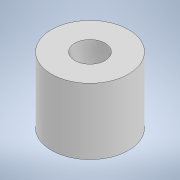
# Autodesk Inventor part: TurnBot
Saved by Autodesk Inventor 2022 (Build 260153000, 153)
## iProperties
Created: 2022-04-06
Part Number: TurnBot
Material: Generic
Document SubType Name: Modeling
Designer: awp
Density: 1 g/cm^3
Appearance: Default
Author: awp
Autodesk Inventor part; units mm, degrees
ref_plane "YZ Plane" through (0, 0, 0) normal (1, 0, 0) x (0, 1, 0)
ref_plane "XZ Plane" through (0, 0, 0) normal (0, 1, 0) x (-1, 0, 0)
ref_plane "XY Plane" through (0, 0, 0) normal (0, 0, 1) x (1, 0, 0)
sketch "Sketch1" plane through (0, 0, 0) normal (0, 1, 0) x (-1, 0, 0)
  circle A0 centre (0, 0) radius 1.975
  circle A1 centre (0, 0) radius 3.5
  line L0 (-2.286, -0.45) -> (2.286, -0.45)
  line L1 (2.286, -0.45) -> (2.286, 0.45)
  line L2 (2.286, 0.45) -> (-2.286, 0.45)
  line L3 (-2.286, 0.45) -> (-2.286, -0.45)
  line L4 (-2.286, -0.45) -> (2.286, 0.45) construction
  line L5 (2.286, -0.45) -> (-2.286, 0.45) construction
  point P0 (-1.9231, 0.45)
  point P1 (1.9231, 0.45)
  point P2 (1.9231, -0.45)
  point P3 (-1.9231, -0.45)
  dimension "d0" = 3.95
  dimension "d1" = 7
  dimension "d2" = 0.9
  dimension "d10" = 4.572
  constraints: 12 end point, 2 centre point, 2 coincident, 2 midpoint, 2 parallel, 1 horizontal, 1 perpendicular
  measures "d0" diameter of A0
  measures "d1" diameter of A1
  measures "d2" distance of L1.end L0.end
  measures "d10" distance of L1.end L2.end
extrude "Extrusion1" add sketch "Sketch1" along normal blind 3 contours A0 L0 L2 | A0 L2 L1 L0 | A0 L0 L3 L2 | A1
sketch "Sketch2" plane through (0, 3, 0) normal (0, 1, 0) x (1, 0, 0)
  circle A0 centre (0, 0) radius 3.5
  constraints: 1 centre point, 1 coincident
extrude "Extrusion2" add sketch "Sketch2" along normal blind 3
sketch "Sketch3" plane through (0, 6, 0) normal (0, 1, 0) x (1, 0, 0)
  circle A0 centre (0, 0) radius 1.375
  dimension "d7" = 2.75
  constraints: 1 centre point, 1 coincident
  measures "d7" diameter of A0
extrude "Extrusion3" cut sketch "Sketch3" against normal blind 3
body "Solid1"
